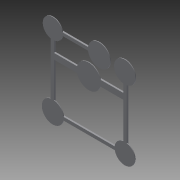
# Autodesk Inventor part: OuterCover
Saved by Autodesk Inventor 2014 SP1 (Build 180222100, 222)
## iProperties
Created: 2014-08-07
Part Number: OuterCover
Material: Generic
Document SubType Name: Modeling
Designer: Erin
Density: 1 g/cm^3
Appearance: Default
Author: Erin
Autodesk Inventor part; units mm, degrees
ref_plane "YZ Plane" through (0, 0, 0) normal (1, 0, 0) x (0, 1, 0)
ref_plane "XZ Plane" through (0, 0, 0) normal (0, 1, 0) x (-1, 0, 0)
ref_plane "XY Plane" through (0, 0, 0) normal (0, 0, 1) x (1, 0, 0)
sketch "Sketch1" plane through (0, 0, 0) normal (0, 1, 0) x (-1, 0, 0)
  line L0 (-31.75, 31.75) -> (31.75, 31.75)
  line L1 (31.75, 31.75) -> (31.75, -31.75)
  line L2 (31.75, -31.75) -> (-31.75, -31.75)
  line L3 (-31.75, -31.75) -> (-31.75, 31.75)
  line L4 (-31.75, 9.25) -> (31.75, 9.25) construction
  line L5 (-31.75, 26.75) -> (-11.75, 26.75) construction
  line L6 (-11.75, 26.75) -> (-11.75, 31.75) construction
  line L7 (32.35, 32.35) -> (-32.35, 32.35)
  line L8 (-32.35, 32.35) -> (-32.35, -32.35)
  line L9 (-32.35, -32.35) -> (32.35, -32.35)
  line L10 (32.35, -32.35) -> (32.35, 32.35)
  line L11 (-35.35, 35.35) -> (35.35, 35.35)
  line L12 (35.35, 35.35) -> (35.35, -35.35)
  line L13 (35.35, -35.35) -> (-35.35, -35.35)
  line L14 (-35.35, -35.35) -> (-35.35, 35.35)
  line L15 (-35.35, 9.25) -> (35.35, 9.25)
  line L16 (35.35, 9.25) -> (35.35, 14.75)
  line L17 (35.35, 14.75) -> (-35.35, 14.75)
  line L18 (-35.35, 14.75) -> (-35.35, 9.25)
  line L19 (-11.75, 31.75) -> (-31.75, 31.75)
  line L20 (-31.75, 31.75) -> (-31.75, 35.35)
  line L21 (-31.75, 35.35) -> (-11.75, 35.35)
  line L22 (-11.75, 35.35) -> (-11.75, 31.75)
  point P0 (0, 0)
  point P1 (0, 31.75)
  point P2 (31.75, 0)
  dimension "d0" = 63.5
  dimension "d1" = 63.5
  dimension "d2" = 41
  dimension "d3" = 5
  dimension "d4" = 20
  dimension "d6" = 3
  dimension "d7" = 0.6
  dimension "d8" = 5.5
  constraints: 46 end point, 11 parallel, 7 perpendicular, 5 point on line, 3 collinear, 3 horizontal, 2 midpoint, 1 horizontal alignment, 1 vertical alignment, 6 other
  measures "d0" distance of L0.start L0.end
  measures "d1" distance of L0.end L1.end
  measures "d2" distance between parallel lines of L2 L4
  measures "d3" distance between parallel lines of L5 L0
  measures "d4" distance of L5.start L5.end
  measures "d6" distance between parallel lines of L7 L11
  measures "d7" distance between parallel lines of L0 L7
  measures "d8" distance between parallel lines of L15 L17
extrude "Extrusion1" add sketch "Sketch1" along normal blind 1.5 contours L17 L1 L15 L3 | L3 L15 L8 L17 | L7 L8 L17 L14 L11 L20 | L22 L11 L12 L17 L10 L7 | L17 L10 L15 L1 | L8 L15 L14 L17 | L8 L9 L10 L15 L12 L13 L14 | L17 L12 L15 L10
sketch "Sketch2" plane through (0, 1.5, 0) normal (0, 1, 0) x (1, 0, 0)
  line L0 (33.5453, -13.8101) -> (-32.898, -13.8101) construction
  line L1 (-32.898, -13.8101) -> (-32.898, -9.1869) construction
  line L2 (-32.898, -9.1869) -> (33.5453, -9.1869) construction
  line L3 (33.5453, -9.1869) -> (33.5453, -13.8101) construction
  line L4 (30.2297, -10.2364) -> (31.1089, -10.2364)
  line L5 (31.1089, -10.2364) -> (31.1089, -11.7878)
  line L6 (31.1089, -11.7878) -> (32.303, -11.7878)
  line L7 (32.303, -11.7878) -> (32.303, -10.2364)
  line L8 (32.303, -10.2364) -> (33.1823, -10.2364)
  line L9 (33.1823, -10.2364) -> (33.1823, -13.7364)
  line L10 (33.1823, -13.7364) -> (32.303, -13.7364)
  line L11 (32.303, -13.7364) -> (32.303, -12.4544)
  line L12 (32.303, -12.4544) -> (31.1089, -12.4544)
  line L13 (31.1089, -12.4544) -> (31.1089, -13.7364)
  line L14 (31.1089, -13.7364) -> (30.2297, -13.7364)
  line L15 (30.2297, -13.7364) -> (30.2297, -10.2364)
  line L16 (29.8808, -10.2364) -> (28.6981, -13.7364)
  line L17 (28.6981, -13.7364) -> (27.7394, -13.7364)
  line L18 (27.7394, -13.7364) -> (26.5567, -10.2364)
  line L19 (26.5567, -10.2364) -> (27.4614, -10.2364)
  line L20 (27.4614, -10.2364) -> (27.6798, -10.9511)
  line L21 (27.6798, -10.9511) -> (28.7803, -10.9511)
  line L22 (28.7803, -10.9511) -> (29.0015, -10.2364)
  line L23 (29.0015, -10.2364) -> (29.8808, -10.2364)
  line L24 (27.8727, -11.5865) -> (28.2301, -12.7437)
  line L25 (28.2301, -12.7437) -> (28.5903, -11.5865)
  line L26 (28.5903, -11.5865) -> (27.8727, -11.5865)
  line L27 (23.2098, -10.2364) -> (24.055, -10.2364)
  line L28 (24.055, -10.2364) -> (25.4051, -12.6756)
  line L29 (25.4051, -12.6756) -> (25.4051, -10.2364)
  line L30 (25.4051, -10.2364) -> (26.2078, -10.2364)
  line L31 (26.2078, -10.2364) -> (26.2078, -13.7364)
  line L32 (26.2078, -13.7364) -> (25.13, -13.7364)
  line L33 (25.13, -13.7364) -> (24.0125, -11.7311)
  line L34 (24.0125, -11.7311) -> (24.0125, -13.7364)
  line L35 (24.0125, -13.7364) -> (23.2098, -13.7364)
  line L36 (23.2098, -13.7364) -> (23.2098, -10.2364)
  spline S0 degree 2 poles (19.3751, -11.9835) (19.3751, -11.4929) (19.8034, -10.7214) (20.1296, -10.5143) knots 0 0 0 1 2 2 2
  spline S1 degree 2 poles (20.1296, -10.5143) (20.4019, -10.3385) (21.0429, -10.2364) (21.4031, -10.2364) knots 0 0 0 1 2 2 2
  line L37 (21.4031, -10.2364) -> (22.4979, -10.2364)
  line L38 (22.4979, -10.2364) -> (22.4979, -13.7364)
  line L39 (22.4979, -13.7364) -> (21.4144, -13.7364)
  spline S2 degree 2 poles (21.4144, -13.7364) (21.0457, -13.7364) (20.4019, -13.6428) (20.1182, -13.4613) knots 0 0 0 1 2 2 2
  spline S3 degree 2 poles (20.1182, -13.4613) (19.775, -13.24) (19.3751, -12.4912) (19.3751, -11.9835) knots 0 0 0 1 2 2 2
  spline S4 degree 2 poles (20.2771, -11.9892) (20.2771, -12.3352) (20.5153, -12.8288) (20.7592, -12.9677) knots 0 0 0 1 2 2 2
  spline S5 degree 2 poles (20.7592, -12.9677) (20.9379, -13.0642) (21.3293, -13.084) (21.6016, -13.084) knots 0 0 0 1 2 2 2
  line L40 (21.6016, -13.084) -> (21.6186, -13.084)
  line L41 (21.6186, -13.084) -> (21.6186, -10.8916)
  line L42 (21.6186, -10.8916) -> (21.6016, -10.8916)
  spline S6 degree 2 poles (21.6016, -10.8916) (21.3067, -10.8916) (20.9011, -10.9114) (20.7167, -11.0277) knots 0 0 0 1 2 2 2
  spline S7 degree 2 poles (20.7167, -11.0277) (20.5011, -11.1639) (20.2771, -11.6432) (20.2771, -11.9892) knots 0 0 0 1 2 2 2
  spline S8 degree 2 poles (14.5222, -10.4349) (14.752, -10.3413) (15.4866, -10.1626) (15.8439, -10.1626) knots 0 0 0 1 2 2 2
  spline S9 degree 2 poles (15.8439, -10.1626) (16.6693, -10.1626) (17.6478, -11.1156) (17.6478, -11.9892) knots 0 0 0 1 2 2 2
  spline S10 degree 2 poles (17.6478, -11.9892) (17.6478, -12.8117) (16.6693, -13.8045) (15.8184, -13.8045) knots 0 0 0 1 2 2 2
  spline S11 degree 2 poles (15.8184, -13.8045) (15.3788, -13.8045) (14.8285, -13.6371) (14.5364, -13.4953) knots 0 0 0 1 2 2 2
  line L43 (14.5364, -13.4953) -> (14.5364, -12.6728)
  line L44 (14.5364, -12.6728) -> (14.6158, -12.6728)
  spline S12 degree 2 poles (14.6158, -12.6728) (14.6782, -12.721) (14.9165, -12.9053) (15.0299, -12.9677) knots 0 0 0 1 2 2 2
  spline S13 degree 2 poles (15.0299, -12.9677) (15.1604, -13.0443) (15.5064, -13.1521) (15.6993, -13.1521) knots 0 0 0 1 2 2 2
  spline S14 degree 2 poles (15.6993, -13.1521) (15.9233, -13.1521) (16.2949, -13.0103) (16.4396, -12.8656) knots 0 0 0 1 2 2 2
  spline S15 degree 2 poles (16.4396, -12.8656) (16.5785, -12.7238) (16.7402, -12.2899) (16.7402, -12.0034) knots 0 0 0 1 2 2 2
  spline S16 degree 2 poles (16.7402, -12.0034) (16.7402, -11.3908) (16.1247, -10.8065) (15.5943, -10.8065) knots 0 0 0 1 2 2 2
  spline S17 degree 2 poles (15.5943, -10.8065) (15.5461, -10.8065) (15.4213, -10.8121) (15.3731, -10.815) knots 0 0 0 1 2 2 2
  line L45 (15.3731, -10.815) -> (15.3731, -11.5042)
  line L46 (15.3731, -11.5042) -> (16.051, -11.5042)
  line L47 (16.051, -11.5042) -> (16.051, -12.1594)
  line L48 (16.051, -12.1594) -> (14.5222, -12.1594)
  line L49 (14.5222, -12.1594) -> (14.5222, -10.4349)
  line L50 (13.8585, -10.2364) -> (13.8585, -13.7364)
  line L51 (13.8585, -13.7364) -> (11.493, -13.7364)
  line L52 (11.493, -13.7364) -> (11.493, -13.0698)
  line L53 (11.493, -13.0698) -> (12.9849, -13.0698)
  line L54 (12.9849, -13.0698) -> (12.9849, -12.4544)
  line L55 (12.9849, -12.4544) -> (11.6093, -12.4544)
  line L56 (11.6093, -12.4544) -> (11.6093, -11.7878)
  line L57 (11.6093, -11.7878) -> (12.9849, -11.7878)
  line L58 (12.9849, -11.7878) -> (12.9849, -10.9029)
  line L59 (12.9849, -10.9029) -> (11.493, -10.9029)
  line L60 (11.493, -10.9029) -> (11.493, -10.2364)
  line L61 (11.493, -10.2364) -> (13.8585, -10.2364)
  spline S18 degree 2 poles (9.8168, -10.174) (10.2195, -10.174) (10.8265, -10.33) (11.0874, -10.4434) knots 0 0 0 1 2 2 2
  line L62 (11.0874, -10.4434) -> (11.0874, -11.2773)
  line L63 (11.0874, -11.2773) -> (11.008, -11.2773)
  spline S19 degree 2 poles (11.008, -11.2773) (10.7443, -11.0532) (10.1118, -10.8121) (9.8139, -10.8121) knots 0 0 0 1 2 2 2
  spline S20 degree 2 poles (9.8139, -10.8121) (9.7374, -10.8121) (9.4906, -10.8462) (9.4169, -10.8802) knots 0 0 0 1 2 2 2
  spline S21 degree 2 poles (9.4169, -10.8802) (9.3261, -10.9199) (9.1985, -11.0646) (9.1985, -11.1809) knots 0 0 0 1 2 2 2
  spline S22 degree 2 poles (9.1985, -11.1809) (9.1985, -11.3142) (9.4055, -11.4787) (9.5473, -11.5156) knots 0 0 0 1 2 2 2
  spline S23 degree 2 poles (9.5473, -11.5156) (9.726, -11.5638) (10.1316, -11.646) (10.3103, -11.7084) knots 0 0 0 1 2 2 2
  spline S24 degree 2 poles (10.3103, -11.7084) (10.7159, -11.8502) (11.0676, -12.3352) (11.0676, -12.6983) knots 0 0 0 1 2 2 2
  spline S25 degree 2 poles (11.0676, -12.6983) (11.0676, -13.189) (10.2366, -13.7988) (9.6126, -13.7988) knots 0 0 0 1 2 2 2
  spline S26 degree 2 poles (9.6126, -13.7988) (9.3006, -13.7988) (8.6823, -13.6711) (8.4383, -13.5634) knots 0 0 0 1 2 2 2
  line L64 (8.4383, -13.5634) -> (8.4383, -12.7635)
  line L65 (8.4383, -12.7635) -> (8.5149, -12.7635)
  spline S27 degree 2 poles (8.5149, -12.7635) (8.7106, -12.9309) (9.2722, -13.1606) (9.5672, -13.1606) knots 0 0 0 1 2 2 2
  spline S28 degree 2 poles (9.5672, -13.1606) (9.6835, -13.1606) (9.865, -13.1266) (9.9671, -13.0812) knots 0 0 0 1 2 2 2
  spline S29 degree 2 poles (9.9671, -13.0812) (10.0494, -13.0443) (10.1685, -12.8968) (10.1685, -12.8061) knots 0 0 0 1 2 2 2
  spline S30 degree 2 poles (10.1685, -12.8061) (10.1685, -12.6699) (9.9785, -12.5139) (9.7062, -12.4515) knots 0 0 0 1 2 2 2
  spline S31 degree 2 poles (9.7062, -12.4515) (9.5303, -12.4118) (9.2041, -12.3352) (9.0169, -12.27) knots 0 0 0 1 2 2 2
  spline S32 degree 2 poles (9.0169, -12.27) (8.6539, -12.1367) (8.2994, -11.6942) (8.2994, -11.3312) knots 0 0 0 1 2 2 2
  spline S33 degree 2 poles (8.2994, -11.3312) (8.2994, -10.8093) (9.1191, -10.174) (9.8168, -10.174) knots 0 0 0 1 2 2 2
  line L66 (7.1762, -10.2364) -> (7.1762, -13.0698)
  line L67 (7.1762, -13.0698) -> (8.2114, -13.0698)
  line L68 (8.2114, -13.0698) -> (8.2114, -13.7364)
  line L69 (8.2114, -13.7364) -> (5.2617, -13.7364)
  line L70 (5.2617, -13.7364) -> (5.2617, -13.0698)
  line L71 (5.2617, -13.0698) -> (6.2969, -13.0698)
  line L72 (6.2969, -13.0698) -> (6.2969, -10.2364)
  line L73 (6.2969, -10.2364) -> (7.1762, -10.2364)
  spline S34 degree 2 poles (3.4862, -10.1626) (4.1924, -10.1626) (4.9525, -10.8433) (4.9525, -11.5014) knots 0 0 0 1 2 2 2
  line L74 (4.9525, -11.5014) -> (4.9525, -13.7364)
  line L75 (4.9525, -13.7364) -> (4.0733, -13.7364)
  line L76 (4.0733, -13.7364) -> (4.0733, -11.5524)
  spline S35 degree 2 poles (4.0733, -11.5524) (4.0733, -11.1865) (3.7981, -10.8292) (3.4862, -10.8292) knots 0 0 0 1 2 2 2
  spline S36 degree 2 poles (3.4862, -10.8292) (3.1827, -10.8292) (2.899, -11.1724) (2.899, -11.5524) knots 0 0 0 1 2 2 2
  line L77 (2.899, -11.5524) -> (2.899, -13.7364)
  line L78 (2.899, -13.7364) -> (2.0198, -13.7364)
  line L79 (2.0198, -13.7364) -> (2.0198, -11.5042)
  spline S37 degree 2 poles (2.0198, -11.5042) (2.0198, -10.8575) (2.7601, -10.1626) (3.4862, -10.1626) knots 0 0 0 1 2 2 2
  line L80 (-1.8886, -10.2364) -> (-0.8194, -10.2364)
  line L81 (-0.8194, -10.2364) -> (0.1535, -11.5212)
  line L82 (0.1535, -11.5212) -> (0.4712, -11.5212)
  line L83 (0.4712, -11.5212) -> (0.4712, -10.2364)
  line L84 (0.4712, -10.2364) -> (1.3447, -10.2364)
  line L85 (1.3447, -10.2364) -> (1.3447, -13.7364)
  line L86 (1.3447, -13.7364) -> (-0.0621, -13.7364)
  spline S38 degree 2 poles (-0.0621, -13.7364) (-0.3542, -13.7364) (-0.7853, -13.6626) (-0.9697, -13.5492) knots 0 0 0 1 2 2 2
  spline S39 degree 2 poles (-0.9697, -13.5492) (-1.1569, -13.4301) (-1.3781, -13.0585) (-1.3781, -12.7749) knots 0 0 0 1 2 2 2
  spline S40 degree 2 poles (-1.3781, -12.7749) (-1.3781, -12.375) (-1.0151, -11.8729) (-0.7116, -11.7254) knots 0 0 0 1 2 2 2
  line L87 (-0.7116, -11.7254) -> (-1.8886, -10.2364)
  spline S41 degree 2 poles (-0.4762, -12.6643) (-0.4762, -12.7976) (-0.3741, -12.9876) (-0.2578, -13.0386) knots 0 0 0 1 2 2 2
  spline S42 degree 2 poles (-0.2578, -13.0386) (-0.1755, -13.0727) (0.0259, -13.0925) (0.1762, -13.0925) knots 0 0 0 1 2 2 2
  line L88 (0.1762, -13.0925) -> (0.4712, -13.0925)
  line L89 (0.4712, -13.0925) -> (0.4712, -12.1509)
  line L90 (0.4712, -12.1509) -> (0.2187, -12.1509)
  spline S43 degree 2 poles (0.2187, -12.1509) (0.0372, -12.1509) (-0.2209, -12.1963) (-0.3088, -12.2672) knots 0 0 0 1 2 2 2
  spline S44 degree 2 poles (-0.3088, -12.2672) (-0.3939, -12.3352) (-0.4762, -12.5168) (-0.4762, -12.6643) knots 0 0 0 1 2 2 2
  line L91 (-2.1496, -10.2364) -> (-2.1496, -13.7364)
  line L92 (-2.1496, -13.7364) -> (-4.5151, -13.7364)
  line L93 (-4.5151, -13.7364) -> (-4.5151, -13.0698)
  line L94 (-4.5151, -13.0698) -> (-3.0232, -13.0698)
  line L95 (-3.0232, -13.0698) -> (-3.0232, -12.4544)
  line L96 (-3.0232, -12.4544) -> (-4.3988, -12.4544)
  line L97 (-4.3988, -12.4544) -> (-4.3988, -11.7878)
  line L98 (-4.3988, -11.7878) -> (-3.0232, -11.7878)
  line L99 (-3.0232, -11.7878) -> (-3.0232, -10.9029)
  line L100 (-3.0232, -10.9029) -> (-4.5151, -10.9029)
  line L101 (-4.5151, -10.9029) -> (-4.5151, -10.2364)
  line L102 (-4.5151, -10.2364) -> (-2.1496, -10.2364)
  spline S45 degree 2 poles (-6.1913, -10.174) (-5.7886, -10.174) (-5.1816, -10.33) (-4.9207, -10.4434) knots 0 0 0 1 2 2 2
  line L103 (-4.9207, -10.4434) -> (-4.9207, -11.2773)
  line L104 (-4.9207, -11.2773) -> (-5.0001, -11.2773)
  spline S46 degree 2 poles (-5.0001, -11.2773) (-5.2638, -11.0532) (-5.8963, -10.8121) (-6.1942, -10.8121) knots 0 0 0 1 2 2 2
  spline S47 degree 2 poles (-6.1942, -10.8121) (-6.2707, -10.8121) (-6.5175, -10.8462) (-6.5912, -10.8802) knots 0 0 0 1 2 2 2
  spline S48 degree 2 poles (-6.5912, -10.8802) (-6.682, -10.9199) (-6.8096, -11.0646) (-6.8096, -11.1809) knots 0 0 0 1 2 2 2
  spline S49 degree 2 poles (-6.8096, -11.1809) (-6.8096, -11.3142) (-6.6026, -11.4787) (-6.4608, -11.5156) knots 0 0 0 1 2 2 2
  spline S50 degree 2 poles (-6.4608, -11.5156) (-6.2821, -11.5638) (-5.8765, -11.646) (-5.6978, -11.7084) knots 0 0 0 1 2 2 2
  spline S51 degree 2 poles (-5.6978, -11.7084) (-5.2922, -11.8502) (-4.9405, -12.3352) (-4.9405, -12.6983) knots 0 0 0 1 2 2 2
  spline S52 degree 2 poles (-4.9405, -12.6983) (-4.9405, -13.189) (-5.7715, -13.7988) (-6.3955, -13.7988) knots 0 0 0 1 2 2 2
  spline S53 degree 2 poles (-6.3955, -13.7988) (-6.7075, -13.7988) (-7.3258, -13.6711) (-7.5698, -13.5634) knots 0 0 0 1 2 2 2
  line L105 (-7.5698, -13.5634) -> (-7.5698, -12.7635)
  line L106 (-7.5698, -12.7635) -> (-7.4932, -12.7635)
  spline S54 degree 2 poles (-7.4932, -12.7635) (-7.2975, -12.9309) (-6.7359, -13.1606) (-6.4409, -13.1606) knots 0 0 0 1 2 2 2
  spline S55 degree 2 poles (-6.4409, -13.1606) (-6.3246, -13.1606) (-6.1431, -13.1266) (-6.041, -13.0812) knots 0 0 0 1 2 2 2
  spline S56 degree 2 poles (-6.041, -13.0812) (-5.9587, -13.0443) (-5.8396, -12.8968) (-5.8396, -12.8061) knots 0 0 0 1 2 2 2
  spline S57 degree 2 poles (-5.8396, -12.8061) (-5.8396, -12.6699) (-6.0297, -12.5139) (-6.3019, -12.4515) knots 0 0 0 1 2 2 2
  spline S58 degree 2 poles (-6.3019, -12.4515) (-6.4778, -12.4118) (-6.804, -12.3352) (-6.9912, -12.27) knots 0 0 0 1 2 2 2
  spline S59 degree 2 poles (-6.9912, -12.27) (-7.3542, -12.1367) (-7.7087, -11.6942) (-7.7087, -11.3312) knots 0 0 0 1 2 2 2
  spline S60 degree 2 poles (-7.7087, -11.3312) (-7.7087, -10.8093) (-6.8891, -10.174) (-6.1913, -10.174) knots 0 0 0 1 2 2 2
  line L107 (-12.6893, -11.4758) -> (-11.4867, -11.4758)
  line L108 (-11.4867, -11.4758) -> (-11.4867, -10.2818)
  line L109 (-11.4867, -10.2818) -> (-10.8656, -10.2818)
  line L110 (-10.8656, -10.2818) -> (-10.8656, -11.4758)
  line L111 (-10.8656, -11.4758) -> (-9.663, -11.4758)
  line L112 (-9.663, -11.4758) -> (-9.663, -12.0828)
  line L113 (-9.663, -12.0828) -> (-10.8656, -12.0828)
  line L114 (-10.8656, -12.0828) -> (-10.8656, -13.2769)
  line L115 (-10.8656, -13.2769) -> (-11.4867, -13.2769)
  line L116 (-11.4867, -13.2769) -> (-11.4867, -12.0828)
  line L117 (-11.4867, -12.0828) -> (-12.6893, -12.0828)
  line L118 (-12.6893, -12.0828) -> (-12.6893, -11.4758)
  line L119 (-15.5908, -10.2364) -> (-15.5908, -13.0698)
  line L120 (-15.5908, -13.0698) -> (-14.5556, -13.0698)
  line L121 (-14.5556, -13.0698) -> (-14.5556, -13.7364)
  line L122 (-14.5556, -13.7364) -> (-17.5053, -13.7364)
  line L123 (-17.5053, -13.7364) -> (-17.5053, -13.0698)
  line L124 (-17.5053, -13.0698) -> (-16.4701, -13.0698)
  line L125 (-16.4701, -13.0698) -> (-16.4701, -10.2364)
  line L126 (-16.4701, -10.2364) -> (-15.5908, -10.2364)
  spline S61 degree 2 poles (-21.0507, -11.9864) (-21.0507, -11.1355) (-20.1431, -10.1626) (-19.3546, -10.1626) knots 0 0 0 1 2 2 2
  spline S62 degree 2 poles (-19.3546, -10.1626) (-18.5633, -10.1626) (-17.6613, -11.1468) (-17.6613, -11.9864) knots 0 0 0 1 2 2 2
  spline S63 degree 2 poles (-17.6613, -11.9864) (-17.6613, -12.8288) (-18.5633, -13.8101) (-19.3546, -13.8101) knots 0 0 0 1 2 2 2
  spline S64 degree 2 poles (-19.3546, -13.8101) (-20.1431, -13.8101) (-21.0507, -12.8344) (-21.0507, -11.9864) knots 0 0 0 1 2 2 2
  spline S65 degree 2 poles (-20.1431, -11.9864) (-20.1431, -12.3012) (-20.0155, -12.7408) (-19.9049, -12.8798) knots 0 0 0 1 2 2 2
  spline S66 degree 2 poles (-19.9049, -12.8798) (-19.7942, -13.0245) (-19.5106, -13.1493) (-19.3574, -13.1493) knots 0 0 0 1 2 2 2
  spline S67 degree 2 poles (-19.3574, -13.1493) (-19.1958, -13.1493) (-18.932, -13.033) (-18.81, -12.8855) knots 0 0 0 1 2 2 2
  spline S68 degree 2 poles (-18.81, -12.8855) (-18.7023, -12.7493) (-18.569, -12.2984) (-18.569, -11.9864) knots 0 0 0 1 2 2 2
  spline S69 degree 2 poles (-18.569, -11.9864) (-18.569, -11.663) (-18.6966, -11.2376) (-18.8072, -11.0929) knots 0 0 0 1 2 2 2
  spline S70 degree 2 poles (-18.8072, -11.0929) (-18.9178, -10.9483) (-19.2043, -10.8235) (-19.3574, -10.8235) knots 0 0 0 1 2 2 2
  spline S71 degree 2 poles (-19.3574, -10.8235) (-19.5134, -10.8235) (-19.8027, -10.9568) (-19.9077, -11.0986) knots 0 0 0 1 2 2 2
  spline S72 degree 2 poles (-19.9077, -11.0986) (-20.0211, -11.2518) (-20.1431, -11.6574) (-20.1431, -11.9864) knots 0 0 0 1 2 2 2
  spline S73 degree 2 poles (-22.9879, -10.1626) (-22.2817, -10.1626) (-21.5215, -10.8433) (-21.5215, -11.5014) knots 0 0 0 1 2 2 2
  line L127 (-21.5215, -11.5014) -> (-21.5215, -13.7364)
  line L128 (-21.5215, -13.7364) -> (-22.4008, -13.7364)
  line L129 (-22.4008, -13.7364) -> (-22.4008, -11.5524)
  spline S74 degree 2 poles (-22.4008, -11.5524) (-22.4008, -11.1865) (-22.6759, -10.8292) (-22.9879, -10.8292) knots 0 0 0 1 2 2 2
  spline S75 degree 2 poles (-22.9879, -10.8292) (-23.2914, -10.8292) (-23.575, -11.1724) (-23.575, -11.5524) knots 0 0 0 1 2 2 2
  line L130 (-23.575, -11.5524) -> (-23.575, -13.7364)
  line L131 (-23.575, -13.7364) -> (-24.4543, -13.7364)
  line L132 (-24.4543, -13.7364) -> (-24.4543, -11.5042)
  spline S76 degree 2 poles (-24.4543, -11.5042) (-24.4543, -10.8575) (-23.714, -10.1626) (-22.9879, -10.1626) knots 0 0 0 1 2 2 2
  spline S77 degree 2 poles (-26.6382, -10.1683) (-25.8497, -10.1683) (-24.9251, -11.1213) (-24.9251, -11.9835) knots 0 0 0 1 2 2 2
  spline S78 degree 2 poles (-24.9251, -11.9835) (-24.9251, -12.8146) (-25.8526, -13.8045) (-26.6411, -13.8045) knots 0 0 0 1 2 2 2
  spline S79 degree 2 poles (-26.6411, -13.8045) (-26.8481, -13.8045) (-27.1828, -13.7562) (-27.336, -13.7165) knots 0 0 0 1 2 2 2
  spline S80 degree 2 poles (-27.336, -13.7165) (-27.4551, -13.6797) (-27.7359, -13.5577) (-27.8238, -13.5123) knots 0 0 0 1 2 2 2
  line L133 (-27.8238, -13.5123) -> (-27.8238, -12.6784)
  line L134 (-27.8238, -12.6784) -> (-27.7359, -12.6784)
  spline S81 degree 2 poles (-27.7359, -12.6784) (-27.6707, -12.7352) (-27.4778, -12.894) (-27.3558, -12.9677) knots 0 0 0 1 2 2 2
  spline S82 degree 2 poles (-27.3558, -12.9677) (-27.2339, -13.0443) (-26.9417, -13.1493) (-26.7801, -13.1493) knots 0 0 0 1 2 2 2
  spline S83 degree 2 poles (-26.7801, -13.1493) (-26.59, -13.1493) (-26.2752, -13.0301) (-26.1305, -12.8798) knots 0 0 0 1 2 2 2
  spline S84 degree 2 poles (-26.1305, -12.8798) (-26.0001, -12.7465) (-25.8327, -12.2899) (-25.8327, -11.9807) knots 0 0 0 1 2 2 2
  spline S85 degree 2 poles (-25.8327, -11.9807) (-25.8327, -11.6545) (-26.0057, -11.2092) (-26.1476, -11.0731) knots 0 0 0 1 2 2 2
  spline S86 degree 2 poles (-26.1476, -11.0731) (-26.2837, -10.9398) (-26.6184, -10.8235) (-26.7857, -10.8235) knots 0 0 0 1 2 2 2
  spline S87 degree 2 poles (-26.7857, -10.8235) (-26.9587, -10.8235) (-27.2736, -10.9398) (-27.3814, -11.0107) knots 0 0 0 1 2 2 2
  spline S88 degree 2 poles (-27.3814, -11.0107) (-27.5005, -11.0816) (-27.6792, -11.2319) (-27.7444, -11.2915) knots 0 0 0 1 2 2 2
  line L135 (-27.7444, -11.2915) -> (-27.8238, -11.2915)
  line L136 (-27.8238, -11.2915) -> (-27.8238, -10.469)
  spline S89 degree 2 poles (-27.8238, -10.469) (-27.7274, -10.4236) (-27.475, -10.3101) (-27.3388, -10.2704) knots 0 0 0 1 2 2 2
  spline S90 degree 2 poles (-27.3388, -10.2704) (-27.1743, -10.2194) (-26.8878, -10.1683) (-26.6382, -10.1683) knots 0 0 0 1 2 2 2
  line L137 (-31.2955, -10.2364) -> (-30.4162, -10.2364)
  line L138 (-30.4162, -10.2364) -> (-30.4162, -11.7878)
  line L139 (-30.4162, -11.7878) -> (-29.2221, -11.7878)
  line L140 (-29.2221, -11.7878) -> (-29.2221, -10.2364)
  line L141 (-29.2221, -10.2364) -> (-28.3429, -10.2364)
  line L142 (-28.3429, -10.2364) -> (-28.3429, -13.7364)
  line L143 (-28.3429, -13.7364) -> (-29.2221, -13.7364)
  line L144 (-29.2221, -13.7364) -> (-29.2221, -12.4544)
  line L145 (-29.2221, -12.4544) -> (-30.4162, -12.4544)
  line L146 (-30.4162, -12.4544) -> (-30.4162, -13.7364)
  line L147 (-30.4162, -13.7364) -> (-31.2955, -13.7364)
  line L148 (-31.2955, -13.7364) -> (-31.2955, -10.2364)
  line L149 (-32.9519, -13.7364) -> (-32.8554, -11.2461)
  line L150 (-32.8554, -11.2461) -> (-32.1123, -11.2461)
  line L151 (-32.1123, -11.2461) -> (-32.0159, -13.7364)
  line L152 (-32.0159, -13.7364) -> (-32.9519, -13.7364)
  line L153 (-32.9462, -10.2364) -> (-32.0215, -10.2364)
  line L154 (-32.0215, -10.2364) -> (-32.0215, -10.8575)
  line L155 (-32.0215, -10.8575) -> (-32.9462, -10.8575)
  line L156 (-32.9462, -10.8575) -> (-32.9462, -10.2364)
  point P0 (0, 0)
  constraints: 2 other
extrude "Extrusion2" add sketch "Sketch2" along normal blind 1
sketch "Sketch3" plane through (0, 0, 0) normal (0, -1, 0) x (1, 0, 0)
  circle A0 centre (-33.5387, 33.85) radius 9.2418
  circle A1 centre (33.55, 32.35) radius 10.0187
  circle A2 centre (-33.5387, -33.4538) radius 10.098
  circle A3 centre (33.55, -33.4538) radius 9.4847
  circle A4 centre (0, 12.057) radius 11.1496
  circle A5 centre (9.6457, 33.85) radius 10.4084
  point P0 (0, 0)
  constraints: 6 centre point
extrude "Extrusion3" add sketch "Sketch3" against normal blind 0.6
body "Solid1"
